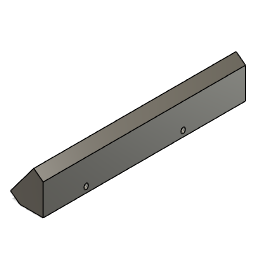
JoyConBody v1 (Autodesk Fusion 360 design; units mm, degrees)
Autodesk Fusion 360 part; units mm, degrees
note: some values were not read from the file. Set by a fixed rule: which sketch regions a step uses.
sketch "スケッチ1" plane through (0, 0, 0) normal (0, 0, 1) x (1, 0, 0)
  line L0 (0, 0) -> (0, 16)
  line L1 (0, 0) -> (-12, 0)
  line L2 (-12, 0) -> (0, 16)
  line L3 (0, 16) -> (0.9, 17.2)
  line L4 (-12, 0) -> (-12.5407, 0)
  line L5 (-12, 0) -> (-12.9, -1.2)
  line L6 (-12, 0) -> (-17.6, 4.2)
  line L7 (-17.6, 4.2) -> (-18.5, 3)
  line L8 (-18.5, 3) -> (-12.9, -1.2)
  line L9 (0, 16) -> (-5.6, 20.2)
  line L10 (-5.6, 20.2) -> (-4.7, 21.4)
  line L11 (-4.7, 21.4) -> (0.9, 17.2)
  line L12 (0.9, 17.2) -> (0.9, -4)
  line L13 (-12.9, -1.2) -> (1.7279, -1.2)
  dimension "d1" = 16
  dimension "d3" = 1.5
  dimension "d4" = 1.5
  dimension "d5" = 7
  dimension "d6" = 1.5
  dimension "d7" = 7
  dimension "d8" = 1.5
  constraint coincident L0.start L1.start
  constraint vertical L0
  constraint perpendicular L0 L1
  constraint parallel L2 L3
  constraint parallel L2 L5
  constraint perpendicular L2 L6
  constraint perpendicular L6 L7
  constraint perpendicular L2 L9
  constraint perpendicular L9 L10
  constraint perpendicular L3 L11
  constraint vertical L12
  constraint perpendicular L12 L13
  measures "d1" distance of L0.start L0.end
  measures "d3" distance of L0.end L3.end
  measures "d4" distance of L1.end L5.end
  measures "d5" distance of L1.end L6.end
  measures "d6" distance of L6.end L7.end
  measures "d7" distance of L0.end L9.end
  measures "d8" distance of L9.end L10.end
extrude "押し出し1" add sketch "スケッチ1" along normal blind 120
sketch "スケッチ2" plane through (-7.68, 5.76, 0) normal (-0.8, 0.6, 0) x (0, 0, 1)
  line L0 (0, 12.8) -> (0, -7.2)
  line L1 (0, -7.2) -> (120, -7.2)
  line L2 (120, -7.2) -> (120, 12.8)
  line L3 (120, 12.8) -> (0, 12.8)
  line L4 (120, 12.8) -> (118.5, 12.8)
  line L5 (118.5, 12.8) -> (118.5, -7.2)
  line L6 (118.5, -7.2) -> (120, -7.2)
  line L7 (120, -7.2) -> (120, 12.8)
  dimension "d11" = 1.5
  dimension "d12" = 20
  constraint horizontal L4
  constraint vertical L5
  constraint horizontal L6
  constraint vertical L7
  constraint coincident L2.end L3.start
  measures "d11" distance of L2.end L4.end
  measures "d12" distance of L2.end L1.end
extrude "押し出し2" add sketch "スケッチ2" along normal blind 7 contours L1 L2 L3 L4 L5 L6 L7
sketch "スケッチ3" plane through (-7.68, 5.76, 0) normal (-0.8, 0.6, 0) x (0, 0, 1)
  line L0 (118.5, -7.2) -> (118.5, 12.8)
  line L1 (118.5, 12.8) -> (0, 12.8)
  line L2 (0, 12.8) -> (0, -7.2)
  line L3 (0, -7.2) -> (118.5, -7.2)
  line L4 (118.5, -7.2) -> (94.5, -7.2)
  line L5 (94.5, -7.2) -> (94.5, 2.3)
  circle A0 centre (94.5, 2.3) radius 1.3
  line L6 (94.5, 2.3) -> (37, 2.3)
  circle A1 centre (37, 2.3) radius 1.3
  dimension "d15" = 24
  dimension "d16" = 9.5
  dimension "d17" = 2.6
  dimension "d18" = 57.5
  dimension "d19" = 2.6
  constraint coincident L0.start L3.end
  constraint perpendicular L0 L4
  constraint perpendicular L4 L5
  constraint coincident L5.end A0.centre
  constraint perpendicular L5 L6
  constraint coincident L6.end A1.centre
  measures "d15" distance of L0.start L4.end
  measures "d16" distance of L4.end L5.end
  measures "d17" diameter of A0
  measures "d18" distance of L5.end L6.end
  measures "d19" diameter of A1
extrude "押し出し3" cut sketch "スケッチ3" against normal blind 20 contours L5 A0 L6 | L5 A0 L6 | A1
sketch "スケッチ4" plane through (-7.68, 5.76, 0) normal (-0.8, 0.6, 0) x (0, 0, 1)
  circle A0 centre (37, 2.3) radius 1.3
  circle A1 centre (94.5, 2.3) radius 1.3
  line L0 (118.5, -7.2) -> (118.5, 12.8)
  line L1 (118.5, 12.8) -> (0, 12.8)
  line L2 (0, 12.8) -> (0, -7.2)
  line L3 (0, -7.2) -> (118.5, -7.2)
  line L4 (0, 12.8) -> (0, 11.8)
  line L5 (0, 11.8) -> (36, 11.8)
  line L6 (36, 11.8) -> (36, 8.8)
  line L7 (36, 8.8) -> (0, 8.8)
  line L8 (0, 8.8) -> (0, 11.8)
  line L9 (0, -7.2) -> (0, -6.2)
  line L10 (0, -6.2) -> (36, -6.2)
  line L11 (36, -6.2) -> (36, -3.2)
  line L12 (36, -3.2) -> (0, -3.2)
  line L13 (0, -3.2) -> (0, -6.2)
  line L14 (36, 11.8) -> (94, 11.8)
  line L15 (36, -6.2) -> (94, -6)
  circle A2 centre (37, 2.3) radius 3.3
  line L16 (40.2999, 2.3211) -> (40.2394, 11.8)
  line L17 (40.2697, 2.7464) -> (40.3005, -6.1852)
  circle A3 centre (94.5, 2.3) radius 3.3
  line L18 (91.2005, 2.2398) -> (91.2305, -6.4364)
  line L19 (91.2005, 2.2398) -> (91.2155, 12.5754)
  dimension "d22" = 1
  dimension "d23" = 3
  dimension "d24" = 1
  dimension "d25" = 3
  dimension "d26" = 2
  dimension "d27" = 2
  constraint coincident L1.end L2.start
  constraint perpendicular L1 L4
  constraint horizontal L5
  constraint vertical L6
  constraint horizontal L7
  constraint vertical L8
  constraint coincident L2.end L3.start
  constraint perpendicular L3 L9
  constraint horizontal L10
  constraint vertical L11
  constraint horizontal L12
  constraint vertical L13
  constraint perpendicular L6 L14
  constraint coincident A2 L16.start
  constraint coincident L14 L16.end
  constraint tangent A2 L16
  constraint coincident A2 L17.start
  constraint coincident L15 L17.end
  constraint perpendicular L15 L17
  constraint coincident A3 L18.start
  constraint perpendicular L15 L18
  measures "d22" distance of L1.end L4.end
  measures "d23" distance of L4.end L7.end
  measures "d24" distance of L2.end L9.end
  measures "d25" distance of L9.end L12.end
extrude "押し出し4" cut sketch "スケッチ4" against normal blind 1 contours L2 L10 L11 L12 L13 | L2 L5 L6 L7 L8 | L14 L15 A2 L16 L17 L18 L19
sketch "スケッチ5" plane through (-7.68, 5.76, 0) normal (-0.8, 0.6, 0) x (0, 0, 1)
  line L0 (36, 8.8) -> (0, 8.8)
  line L1 (0, 8.8) -> (0, -3.2)
  line L2 (0, -3.2) -> (36, -3.2)
  line L3 (36, -3.2) -> (36, -6.2)
  line L4 (36, -6.2) -> (0, -6.2)
  line L5 (0, -6.2) -> (0, -7.2)
  line L6 (0, -7.2) -> (118.5, -7.2)
  line L7 (118.5, -7.2) -> (118.5, 12.8)
  line L8 (118.5, 12.8) -> (0, 12.8)
  line L9 (0, 12.8) -> (0, 11.8)
  line L10 (0, 11.8) -> (36, 11.8)
  line L11 (36, 11.8) -> (36, 8.8)
  line L12 (40.2394, 11.8) -> (91.2144, 11.8)
  line L13 (91.2144, 11.8) -> (91.2007, 2.3697)
  arc A0 (91.2007, 2.3697) -> (91.2005, 2.2398) centre (94.5, 2.3) ccw
  line L14 (91.2005, 2.2398) -> (91.229, -6.0096)
  line L15 (91.229, -6.0096) -> (40.3005, -6.1852)
  line L16 (40.3005, -6.1852) -> (40.2727, 1.8761)
  arc A1 (40.2727, 1.8761) -> (40.2999, 2.3211) centre (37, 2.3) ccw
  line L17 (40.2999, 2.3211) -> (40.2394, 11.8)
  circle A2 centre (37, 2.3) radius 1.3
  circle A3 centre (94.5, 2.3) radius 1.3
  line L18 (37, 11.8) -> (37, 7.8)
  line L19 (37, 7.8) -> (1, 7.8)
  line L20 (1, 7.8) -> (1, -2.2)
  line L21 (1, -2.2) -> (37, -2.2)
  line L22 (37, -2.2) -> (37, -6.2)
  line L23 (37, -6.2) -> (117.5, -6.2)
  line L24 (117.5, -6.2) -> (117.5, 11.8)
  line L25 (117.5, 11.8) -> (37, 11.8)
  line L26 (101.4988, 11.8) -> (101.4988, -6.2)
  dimension "d30" = -1
  constraint coincident L25 L26.start
  constraint coincident L23 L26.end
  constraint perpendicular L23 L26
extrude "押し出し5" cut sketch "スケッチ5" against normal blind 1 contours L23 L24 L25 L26
